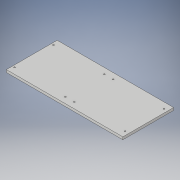
# Autodesk Inventor part: 4326electronicsboard
Saved by Autodesk Inventor 2019 (Build 230136000, 136)
## iProperties
Created: 2019-10-23
Part Number: 4326electronicsboard
Material: Generic
Document SubType Name: Modeling
Designer: shrey
Density: 1 g/cm^3
Appearance: Default
Author: shrey
Autodesk Inventor part; units mm, degrees
ref_plane "YZ Plane" through (0, 0, 0) normal (1, 0, 0) x (0, 1, 0)
ref_plane "XZ Plane" through (0, 0, 0) normal (0, 1, 0) x (-1, 0, 0)
ref_plane "XY Plane" through (0, 0, 0) normal (0, 0, 1) x (1, 0, 0)
sketch "Sketch1" plane through (0, 0, 0) normal (0, 1, 0) x (-1, 0, 0)
  line L0 (146.685, 64) -> (-146.685, 64)
  line L1 (-146.685, 64) -> (-146.685, -64)
  line L2 (-146.685, -64) -> (146.685, -64)
  line L3 (146.685, -64) -> (146.685, 64)
  line L4 (146.685, 64) -> (-146.685, -64) construction
  line L5 (-146.685, 64) -> (146.685, -64) construction
  line L6 (0, 0) -> (1.8415, 0) construction
  line L7 (144.8415, 0) -> (144.8415, -44) construction
  line L8 (144.8415, -44) -> (1.8415, -44) construction
  line L9 (1.8415, -44) -> (1.8415, 0) construction
  line L10 (144.8415, 0) -> (144.8415, 44) construction
  line L11 (144.8415, 44) -> (1.8415, 44) construction
  line L12 (1.8415, 44) -> (1.8415, 0) construction
  line L13 (-146.685, 64) -> (146.685, -64) construction
  line L14 (-144.8415, 0) -> (-144.8415, 51.5) construction
  line L15 (-144.8415, 51.5) -> (-1.8415, 51.5) construction
  line L16 (-1.8415, 51.5) -> (-1.8415, 0) construction
  line L17 (144.8415, -44) -> (137.3415, -44) construction
  line L18 (137.3415, -41.5) -> (144.8415, -41.5) construction
  line L19 (144.8415, -41.5) -> (144.8415, -44) construction
  line L20 (1.8415, -44) -> (9.3415, -44) construction
  line L21 (9.3415, -41.5) -> (1.8415, -41.5) construction
  line L22 (-1.8415, 0) -> (-144.8415, 0) construction
  line L23 (-144.8415, 0) -> (-144.8415, -51.5) construction
  line L24 (-144.8415, -51.5) -> (-1.8415, -51.5) construction
  line L25 (-1.8415, -51.5) -> (-1.8415, 0) construction
  line L26 (-1.8415, 51.5) -> (-9.3415, 51.5) construction
  line L27 (-9.3415, 51.5) -> (-9.3415, 49) construction
  line L28 (-9.3415, 49) -> (-1.8415, 49) construction
  line L29 (-1.8415, 49) -> (-1.8415, 51.5) construction
  circle A0 centre (-9.3415, 49) radius 1.7
  line L30 (-144.8415, 51.5) -> (-137.3415, 51.5) construction
  line L31 (-137.3415, 51.5) -> (-137.3415, 49) construction
  line L32 (-137.3415, 49) -> (-144.8415, 49) construction
  line L33 (-144.8415, 49) -> (-144.8415, 51.5) construction
  circle A1 centre (-137.3415, 49) radius 1.7
  circle A2 centre (-9.3415, -49) radius 1.7
  circle A3 centre (-137.3415, -49) radius 1.7
  circle A4 centre (13.0245, 49) radius 1.7
  circle A5 centre (141.0245, 49) radius 1.7
  circle A6 centre (13.0245, -49) radius 1.7
  circle A7 centre (141.0245, -49) radius 1.7
  dimension "d0" = 293.37
  dimension "d1" = 128
  dimension "d2" = 1.8415
  dimension "d3" = 143
  dimension "d4" = 44
  dimension "d5" = 7.5
  dimension "d8" = 7.5
  dimension "d14" = 51.5
  dimension "d15" = 143
  dimension "d16" = 51.5
  dimension "d17" = 7.5
  dimension "d18" = 2.5
  dimension "d19" = 3.4
  dimension "d20" = 7.5
  dimension "d21" = 2.5
  dimension "d22" = 3.4
  constraints: 68 end point, 11 parallel, 8 centre point, 7 horizontal, 6 symmetric about line, 4 perpendicular, 2 coincident, 2 midpoint, 6 other
  measures "d0" distance of L1.end L2.end
  measures "d1" distance of L0.end L1.end
  measures "d2" distance of L6.start L6.end
  measures "d3" distance of L6.end L7.start
  measures "d4" distance of L7.start L7.end
  measures "d5" distance of L18.start L18.end
  measures "d8" distance of L21.end L21.start
  measures "d14" distance of L14.start L15.start
  measures "d15" distance of L24.end L23.end
  measures "d16" distance of L23.end L22.end
  measures "d17" distance of L28.end L27.end
  measures "d18" distance of L27.end L26.end
  measures "d19" diameter of A0
  measures "d20" distance of L31.end L32.end
  measures "d21" distance of L30.end L31.end
  measures "d22" diameter of A1
extrude "Extrusion2" add sketch "Sketch1" along normal blind 6.35
body "Solid2"
